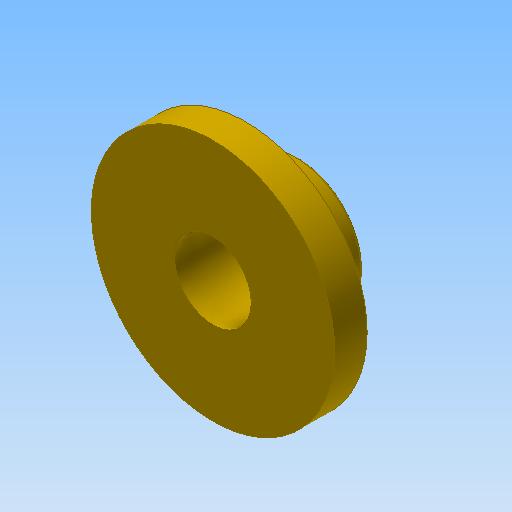
# Autodesk Inventor part: XL200 PART2
Saved by Autodesk Inventor 2020.1 (Build 241239000, 239)
## iProperties
Created: 2001-03-07
Part Number: XL200 PART2
Document SubType Name: Modeling
Designer: Joe M
Material: Steel, Mild
Engineer: Joe M
Density: 7.86 g/cm^3
Appearance: Mastenbroek
Control State: 0
Master: False
Checked Out: False
Shininess: 20.0
Length Units: 11269
Angle Units: 11279
Time Units: 11290
Mass Units: 11283
Length Display Precision: 3
Angle Display Precision: 2
Compacted: True
Density: 0.0
Volumn: 0.0
Area: 0.0
PropertySet Name: Model Information
Author: Joe M
Autodesk Inventor part; units mm, degrees
ref_plane "YZ Plane" through (0, 0, 0) normal (1, 0, 0) x (0, 1, 0)
ref_plane "XZ Plane" through (0, 0, 0) normal (0, 1, 0) x (-1, 0, 0)
ref_plane "XY Plane" through (0, 0, 0) normal (0, 0, 1) x (1, 0, 0)
sketch "Sketch1" plane through (-96.571, 93.5084, -10) normal (0, 0, 1) x (1, 0, 0)
  circle A0 centre (96.571, -93.5084) radius 75
  dimension "d15" = 150
  constraints: 1 centre point, 1 other
  measures "d15" diameter of A0
extrude "ExtrusionBlind1" add sketch "Sketch1" along normal blind 20
sketch "Sketch2" plane through (-96.571, 93.5084, -10) normal (0, 0, 1) x (1, 0, 0)
  circle A0 centre (96.571, -93.5084) radius 40
  circle A1 centre (96.571, -93.5084) radius 75 projected
  dimension "d16" = 80
  constraints: 1 centre point, 1 concentric
  measures "d16" diameter of A0
extrude "ExtrusionBlind2" add sketch "Sketch2" against normal blind 33 contours A0
chamfer "Chamfer1" distance 33 angle 15 1 edges at (-40, 0, -10) measured on face at (-40, 0, -10.5)
fillet "Fillet1" radius 3 3 edges at (-48.8422, 0, -10) (-40, 0, -42.9999) (-40, 0, -43)
sketch "Sketch3" plane through (0, 0, -43) normal (0, 0, -1) x (-1, 0, 0)
  circle A0 centre (0, 0) radius 48.2465 projected
  point P0 (0, 0)
hole "Hole1" at (0, 0, -43) direction (0, 0, 1) diameter 47.2 end through all
body "Solid1"
